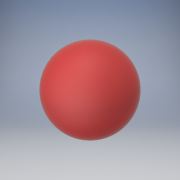
# Autodesk Inventor part: Sphère
Saved by Autodesk Inventor 2019.3 (Build 233278000, 278)
## iProperties
Created: 2019-03-04
Part Number: Sphère
Material: Plastique ABS
Document SubType Name: Modeling
Designer: Houba Guillaume
Mass: 35.5209 g
Surface Area: 50.2655 cm^2
Volume: 33.5103 cm^3
Density: 1.06 g/cm^3
Appearance: Lisse - Rouge
Author: Houba Guillaume
## iProperties of the stored document Sphère_Impression 3D.ipt
Created: 2019-03-04
Part Number: Sphère_Impression 3D
Material: Générique
Document SubType Name: Modeling
Designer: Houba Guillaume
Mass: 33.5103 g
Surface Area: 50.2655 cm^2
Volume: 33.5103 cm^3
Density: 1 g/cm^3
Appearance: Par défaut
Author: Houba Guillaume
Autodesk Inventor part; units mm, degrees
ref_plane "YZ Plane" through (0, 0, 0) normal (1, 0, 0) x (0, 1, 0)
ref_plane "XZ Plane" through (0, 0, 0) normal (0, 1, 0) x (-1, 0, 0)
ref_plane "XY Plane" through (0, 0, 0) normal (0, 0, 1) x (1, 0, 0)
sketch "Esquisse1" plane through (0, 0, 0) normal (0, 1, 0) x (-1, 0, 0)
  line L0 (0, -12.7) -> (0, 27.3)
  arc A0 (0, 27.3) -> (0, -12.7) centre (0, 7.3) ccw
  line L1 (25.4, 7.3) -> (-25.4, 7.3) construction
  dimension "d0" = 40
  constraints: 4 end point, 2 midpoint, 2 point on circle, 1 centre point, 1 coincident, 1 perpendicular, 1 vertical
  measures "d0" distance of L0.start L0.end
revolve "Sphère1" add sketch "Esquisse1" angle 360 about axis through (0, 0, -12.7) along (0, 0, 1)
equation "\"d0\" = dd0"
equation "\"dd0\" = 40"
